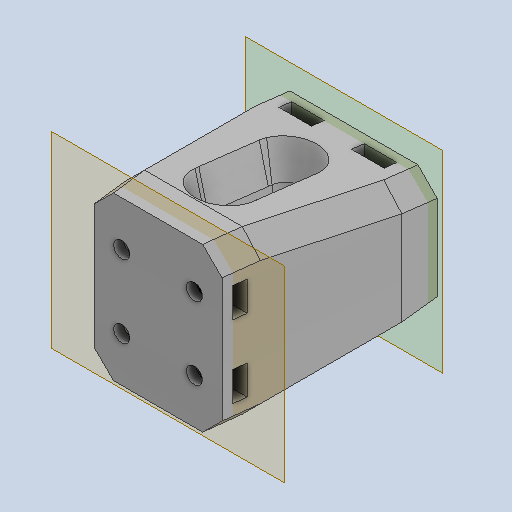
# Autodesk Inventor part: MCP-I
Saved by Autodesk Inventor 2026 (Build 300175050, 175E)
## iProperties
Created: 2025-12-08
Part Number: MCP-I
Material: Genérico
Document SubType Name: Modeling
Designer: user
Density: 1 g/cm^3
Appearance: Gris claro
Mass: 12.7013 g
Surface Area: 55.8888 cm^2
Volume: 12.7013 cm^3
Author: user
Autodesk Inventor part; units mm, degrees
ref_plane "YZ Plane" through (0, 0, 0) normal (1, 0, 0) x (0, 1, 0)
ref_plane "XZ Plane" through (0, 0, 0) normal (0, 1, 0) x (-1, 0, 0)
ref_plane "XY Plane" through (0, 0, 0) normal (0, 0, 1) x (1, 0, 0)
sketch "Boceto1" plane through (0, 0, 0) normal (0, 0, 1) x (1, 0, 0)
  line L0 (-9.8, -13.3) -> (-9.8, 13.3) construction
  line L1 (9.8, 13.3) -> (-9.8, 13.3) construction
  line L2 (9.8, 13.3) -> (9.8, -13.3) construction
  line L3 (-9.8, -13.3) -> (9.8, -13.3) construction
  circle A0 centre (-8, -8) radius 0.8 construction
  circle A1 centre (8, 8) radius 0.8 construction
  circle A2 centre (-8, 8) radius 0.8 construction
  circle A3 centre (0, 0) radius 4 construction
  circle A4 centre (0, -6) radius 1.025 construction
  circle A5 centre (-6, 0) radius 1.025 construction
  circle A6 centre (0, 6) radius 1.025 construction
  circle A7 centre (6, 0) radius 1.025 construction
  circle A8 centre (-5.6569, -5.6569) radius 1.025 construction
  circle A9 centre (-5.6569, 5.6569) radius 1.025 construction
  circle A10 centre (5.6569, 5.6569) radius 1.025 construction
  circle A11 centre (5.6569, -5.6569) radius 1.025 construction
  circle A12 centre (3, -9) radius 1.025 construction
  circle A13 centre (-3, -9) radius 1.025 construction
  circle A14 centre (3, 9) radius 1.025 construction
  circle A15 centre (-3, 9) radius 1.025 construction
  circle A16 centre (8, -8) radius 0.8 construction
  circle A17 centre (5.6569, 5.6569) radius 1.25
  circle A18 centre (5.6569, -5.6569) radius 1.25
  circle A19 centre (-5.6569, -5.6569) radius 1.25
  circle A20 centre (-5.6569, 5.6569) radius 1.25
  line L4 (16.5, -9.7) -> (16.5, 9.7) construction
  line L5 (16.5, 9.7) -> (-16.5, 9.7) construction
  line L6 (-16.5, -9.7) -> (16.5, -9.7) construction
  line L7 (-16.5, -9.7) -> (-16.5, 9.7) construction
  arc A21 (3.8297, -1.1547) -> (3.8297, 1.1547) centre (0, 0) ccw construction
  line L8 (3.8297, -1.1547) -> (4, -1.1547) construction
  line L9 (4, -1.1547) -> (4.7835, -1.6071) construction
  line L10 (4.7835, -1.6071) -> (4.8435, -1.5031) construction
  line L11 (4.8435, -1.5031) -> (5.2765, -1.7531) construction
  line L12 (5.2765, -1.7531) -> (5.2165, -1.8571) construction
  line L13 (5.2165, -1.8571) -> (6, -2.3094) construction
  line L14 (6, -2.3094) -> (8, -1.1547) construction
  line L15 (8, -1.1547) -> (8, -0.25) construction
  line L16 (8, -0.25) -> (7.88, -0.25) construction
  line L17 (7.88, -0.25) -> (7.88, 0.25) construction
  line L18 (7.88, 0.25) -> (8, 0.25) construction
  line L19 (8, 0.25) -> (8, 1.1547) construction
  line L20 (8, 1.1547) -> (6, 2.3094) construction
  line L21 (6, 2.3094) -> (5.2165, 1.8571) construction
  line L22 (5.2165, 1.8571) -> (5.2765, 1.7531) construction
  line L23 (5.2765, 1.7531) -> (4.8435, 1.5031) construction
  line L24 (4.8435, 1.5031) -> (4.7835, 1.6071) construction
  line L25 (4.7835, 1.6071) -> (4, 1.1547) construction
  line L26 (4, 1.1547) -> (3.8297, 1.1547) construction
  circle A22 centre (6, 0) radius 1.025 construction
  arc A23 (3.8297, -1.1547) -> (3.8297, 1.1547) centre (0, 0) ccw construction
  line L27 (3.8297, -1.1547) -> (4, -1.1547) construction
  line L28 (4, -1.1547) -> (4.7835, -1.6071) construction
  line L29 (4.7835, -1.6071) -> (4.8435, -1.5031) construction
  line L30 (4.8435, -1.5031) -> (5.2765, -1.7531) construction
  line L31 (5.2765, -1.7531) -> (5.2165, -1.8571) construction
  line L32 (5.2165, -1.8571) -> (6, -2.3094) construction
  line L33 (6, -2.3094) -> (8, -1.1547) construction
  line L34 (8, -1.1547) -> (8, -0.25) construction
  line L35 (8, -0.25) -> (7.88, -0.25) construction
  line L36 (7.88, -0.25) -> (7.88, 0.25) construction
  line L37 (7.88, 0.25) -> (8, 0.25) construction
  line L38 (8, 0.25) -> (8, 1.1547) construction
  line L39 (8, 1.1547) -> (6, 2.3094) construction
  line L40 (6, 2.3094) -> (5.2165, 1.8571) construction
  line L41 (5.2165, 1.8571) -> (5.2765, 1.7531) construction
  line L42 (5.2765, 1.7531) -> (4.8435, 1.5031) construction
  line L43 (4.8435, 1.5031) -> (4.7835, 1.6071) construction
  line L44 (4.7835, 1.6071) -> (4, 1.1547) construction
  line L45 (4, 1.1547) -> (3.8297, 1.1547) construction
  circle A24 centre (6, 0) radius 1.025 construction
  line L46 (3.3475, 5.6569) -> (4.5022, 7.6569) construction
  line L47 (4.5022, 7.6569) -> (6.8116, 7.6569) construction
  line L48 (6.8116, 7.6569) -> (7.9663, 5.6569) construction
  line L49 (7.9663, 5.6569) -> (6.8116, 3.6569) construction
  line L50 (6.8116, 3.6569) -> (4.5022, 3.6569) construction
  line L51 (4.5022, 3.6569) -> (3.3475, 5.6569) construction
  line L52 (12.9663, -12.6569) -> (-12.9663, -12.6569)
  line L53 (-12.9663, -12.6569) -> (-12.9663, 12.6569)
  line L54 (-12.9663, 12.6569) -> (12.9663, 12.6569)
  line L55 (12.9663, 12.6569) -> (12.9663, -12.6569)
  line L56 (12.9663, -12.6569) -> (-12.9663, 12.6569) construction
  line L57 (-12.9663, -12.6569) -> (12.9663, 12.6569) construction
  line L58 (3.6569, -4.5022) -> (5.6569, -3.3475) construction
  line L59 (5.6569, -3.3475) -> (7.6569, -4.5022) construction
  line L60 (7.6569, -4.5022) -> (7.6569, -6.8116) construction
  line L61 (7.6569, -6.8116) -> (5.6569, -7.9663) construction
  line L62 (5.6569, -7.9663) -> (3.6569, -6.8116) construction
  line L63 (3.6569, -6.8116) -> (3.6569, -4.5022) construction
  point P0 (0, 0)
  point P1 (9.8, -9.7)
  point P2 (9.8, 9.7)
  point P3 (-9.8, -9.7)
  point P4 (-9.8, 9.7)
  point P5 (16.5, 9.7)
extrude "Extrusión1" add sketch "Boceto1" along normal mid plane 30.507
ref_plane "Plano de trabajo1" through (0, 0, 13.7535) normal (0, 0, 1) x (1, 0, 0)
sketch "Boceto2" plane through (0, 0, 13.7535) normal (0, 0, -1) x (-1, 0, 0)
  circle A0 centre (-5.6569, 5.6569) radius 1.25 projected
  circle A1 centre (-5.6569, -5.6569) radius 1.25 projected
  circle A2 centre (5.6569, -5.6569) radius 1.25 projected
  circle A3 centre (5.6569, 5.6569) radius 1.25 projected
  line L0 (-12.9663, 12.6569) -> (-12.9663, -12.6569) projected
  line L1 (-12.9663, -12.6569) -> (12.9663, -12.6569) projected
  line L2 (12.9663, -12.6569) -> (12.9663, 12.6569) projected
  line L3 (12.9663, 12.6569) -> (-12.9663, 12.6569) projected
  arc A4 (-3.8297, 1.1547) -> (-3.8297, -1.1547) centre (0, 0) ccw construction
  line L4 (-3.8297, -1.1547) -> (-4, -1.1547) construction
  line L5 (-4, -1.1547) -> (-4.7835, -1.6071) construction
  line L6 (-4.7835, -1.6071) -> (-4.8435, -1.5031) construction
  line L7 (-4.8435, -1.5031) -> (-5.2765, -1.7531) construction
  line L8 (-5.2765, -1.7531) -> (-5.2165, -1.8571) construction
  line L9 (-5.2165, -1.8571) -> (-6, -2.3094) construction
  line L10 (-6, -2.3094) -> (-8, -1.1547) construction
  line L11 (-8, -1.1547) -> (-8, -0.25) construction
  line L12 (-8, -0.25) -> (-7.88, -0.25) construction
  line L13 (-7.88, -0.25) -> (-7.88, 0.25) construction
  line L14 (-7.88, 0.25) -> (-8, 0.25) construction
  line L15 (-8, 0.25) -> (-8, 1.1547) construction
  line L16 (-8, 1.1547) -> (-6, 2.3094) construction
  line L17 (-6, 2.3094) -> (-5.2165, 1.8571) construction
  line L18 (-5.2165, 1.8571) -> (-5.2765, 1.7531) construction
  line L19 (-5.2765, 1.7531) -> (-4.8435, 1.5031) construction
  line L20 (-4.8435, 1.5031) -> (-4.7835, 1.6071) construction
  line L21 (-4.7835, 1.6071) -> (-4, 1.1547) construction
  line L22 (-4, 1.1547) -> (-3.8297, 1.1547) construction
  circle A5 centre (-6, 0) radius 1.025 construction
  line L23 (-3.6569, -6.8116) -> (-5.6569, -7.9663)
  line L24 (-5.6569, -7.9663) -> (-7.6569, -6.8116)
  line L25 (-7.6569, -6.8116) -> (-7.6569, -4.5022)
  line L26 (-7.6569, -4.5022) -> (-5.6569, -3.3475)
  line L27 (-5.6569, -3.3475) -> (-3.6569, -4.5022)
  line L28 (-3.6569, -4.5022) -> (-3.6569, -6.8116)
  line L29 (-5.6569, -7.9663) -> (-12.9663, -7.9663)
  line L30 (-12.9663, -7.9663) -> (-12.9663, -3.3475)
  line L31 (-12.9663, -3.3475) -> (-5.6569, -3.3475)
  line L32 (-12.9663, 0) -> (12.9663, 0) construction
  line L33 (0, -12.6569) -> (0, 12.6569) construction
  circle A6 centre (-5.6569, 5.6569) radius 1.25
  line L34 (-3.6569, 6.8116) -> (-5.6569, 7.9663)
  line L35 (-5.6569, 7.9663) -> (-7.6569, 6.8116)
  line L36 (-7.6569, 6.8116) -> (-7.6569, 4.5022)
  line L37 (-7.6569, 4.5022) -> (-5.6569, 3.3475)
  line L38 (-5.6569, 3.3475) -> (-3.6569, 4.5022)
  line L39 (-3.6569, 4.5022) -> (-3.6569, 6.8116)
  line L40 (-5.6569, 7.9663) -> (-12.9663, 7.9663)
  line L41 (-12.9663, 7.9663) -> (-12.9663, 3.3475)
  line L42 (-12.9663, 3.3475) -> (-5.6569, 3.3475)
  circle A7 centre (5.6569, 5.6569) radius 1.25
  circle A8 centre (5.6569, -5.6569) radius 1.25
  line L43 (3.6569, -6.8116) -> (5.6569, -7.9663)
  line L44 (5.6569, -7.9663) -> (7.6569, -6.8116)
  line L45 (7.6569, -6.8116) -> (7.6569, -4.5022)
  line L46 (7.6569, -4.5022) -> (5.6569, -3.3475)
  line L47 (5.6569, -3.3475) -> (3.6569, -4.5022)
  line L48 (3.6569, -4.5022) -> (3.6569, -6.8116)
  line L49 (5.6569, -7.9663) -> (12.9663, -7.9663)
  line L50 (12.9663, -7.9663) -> (12.9663, -3.3475)
  line L51 (12.9663, -3.3475) -> (5.6569, -3.3475)
  circle A9 centre (5.6569, 5.6569) radius 1.25
  line L52 (7.6569, 4.5022) -> (5.6569, 3.3475)
  line L53 (5.6569, 3.3475) -> (3.6569, 4.5022)
  line L54 (7.6569, 6.8116) -> (7.6569, 4.5022)
  line L55 (3.6569, 4.5022) -> (3.6569, 6.8116)
  line L56 (3.6569, 6.8116) -> (5.6569, 7.9663)
  line L57 (5.6569, 7.9663) -> (7.6569, 6.8116)
  line L58 (12.9663, 3.3475) -> (5.6569, 3.3475)
  line L59 (12.9663, 7.9663) -> (12.9663, 3.3475)
  line L60 (5.6569, 7.9663) -> (12.9663, 7.9663)
  dimension "d120" = 4.6188
  dimension "d121" = 4.6188
  constraints: 76 end point, 31 symmetric about line, 4 centre point, 4 coincident, 4 midpoint, 2 parallel, 2 perpendicular, 2 vertical, 1 collinear, 1 horizontal, 17 other
  measures "d120" distance of L16.end L9.end
  measures "d121" distance of L26.end L23.end
extrude "Extrusión2" cut sketch "Boceto2" along normal blind 2 contours A0 | A1 | A2 | A3 | L40 L35 L36 L37 L42 L0 | L34 L39 L38 L37 L36 L35 | L2 L58 L52 L54 L57 L60 | L31 L26 L25 L24 L29 L0 | L57 L54 L52 L53 L55 L56 | L27 L28 L23 L24 L25 L26 | L2 L49 L44 L45 L46 L51 | L46 L45 L44 L43 L48 L47
mirror "Simetría2" [suppressed]
ref_plane "Plano de trabajo2" through (0, 0, -13.7535) normal (0, 0, -1) x (-1, 0, 0)
sketch "Boceto7" plane through (0, 0, -13.7535) normal (0, 0, -1) x (-1, 0, 0)
  circle A0 centre (-5.6569, 5.6569) radius 1.25 projected
  circle A1 centre (-5.6569, -5.6569) radius 1.25 projected
  circle A2 centre (5.6569, -5.6569) radius 1.25 projected
  circle A3 centre (5.6569, 5.6569) radius 1.25 projected
  line L0 (-12.9663, -12.6569) -> (-12.9663, 12.6569) projected
  line L1 (-12.9663, 12.6569) -> (12.9663, 12.6569) projected
  line L2 (12.9663, 12.6569) -> (12.9663, -12.6569) projected
  line L3 (12.9663, -12.6569) -> (-12.9663, -12.6569) projected
  arc A4 (-1.1547, -3.8297) -> (1.1547, -3.8297) centre (0, 0) ccw construction
  line L4 (-1.1547, -3.8297) -> (-1.1547, -4) construction
  line L5 (-1.1547, -4) -> (-1.6071, -4.7835) construction
  line L6 (-1.6071, -4.7835) -> (-1.5031, -4.8435) construction
  line L7 (-1.5031, -4.8435) -> (-1.7531, -5.2765) construction
  line L8 (-1.7531, -5.2765) -> (-1.8571, -5.2165) construction
  line L9 (-1.8571, -5.2165) -> (-2.3094, -6) construction
  line L10 (-2.3094, -6) -> (-1.1547, -8) construction
  line L11 (-1.1547, -8) -> (-0.25, -8) construction
  line L12 (-0.25, -8) -> (-0.25, -7.88) construction
  line L13 (-0.25, -7.88) -> (0.25, -7.88) construction
  line L14 (0.25, -7.88) -> (0.25, -8) construction
  line L15 (0.25, -8) -> (1.1547, -8) construction
  line L16 (1.1547, -8) -> (2.3094, -6) construction
  line L17 (2.3094, -6) -> (1.8571, -5.2165) construction
  line L18 (1.8571, -5.2165) -> (1.7531, -5.2765) construction
  line L19 (1.7531, -5.2765) -> (1.5031, -4.8435) construction
  line L20 (1.5031, -4.8435) -> (1.6071, -4.7835) construction
  line L21 (1.6071, -4.7835) -> (1.1547, -4) construction
  line L22 (1.1547, -4) -> (1.1547, -3.8297) construction
  circle A5 centre (0, -6) radius 1.025 construction
  line L23 (4.5022, -7.6569) -> (3.3475, -5.6569) construction
  line L24 (3.3475, -5.6569) -> (4.5022, -3.6569) construction
  line L25 (4.5022, -3.6569) -> (6.8116, -3.6569) construction
  line L26 (6.8116, -3.6569) -> (7.9663, -5.6569) construction
  line L27 (7.9663, -5.6569) -> (6.8116, -7.6569) construction
  line L28 (6.8116, -7.6569) -> (4.5022, -7.6569) construction
  line L29 (4.3867, -7.8569) -> (3.1165, -5.6569)
  line L30 (3.1165, -5.6569) -> (4.3867, -3.4569)
  line L31 (4.3867, -3.4569) -> (6.927, -3.4569)
  line L32 (6.927, -3.4569) -> (8.1972, -5.6569)
  line L33 (8.1972, -5.6569) -> (6.927, -7.8569)
  line L34 (6.927, -7.8569) -> (4.3867, -7.8569)
  line L35 (3.1165, -5.6569) -> (3.1165, -12.6569)
  line L36 (3.1165, -12.6569) -> (8.1972, -12.6569)
  line L37 (8.1972, -12.6569) -> (8.1972, -5.6569)
  line L38 (12.9663, 0) -> (-12.9663, 0) construction
  line L39 (0, 12.6569) -> (0, -12.6569) construction
  circle A6 centre (5.6569, 5.6569) radius 1.25
  line L40 (4.5022, 7.6569) -> (3.3475, 5.6569) construction
  line L41 (3.3475, 5.6569) -> (4.5022, 3.6569) construction
  line L42 (4.5022, 3.6569) -> (6.8116, 3.6569) construction
  line L43 (6.8116, 3.6569) -> (7.9663, 5.6569) construction
  line L44 (7.9663, 5.6569) -> (6.8116, 7.6569) construction
  line L45 (6.8116, 7.6569) -> (4.5022, 7.6569) construction
  line L46 (4.3867, 7.8569) -> (3.1165, 5.6569)
  line L47 (3.1165, 5.6569) -> (4.3867, 3.4569)
  line L48 (4.3867, 3.4569) -> (6.927, 3.4569)
  line L49 (6.927, 3.4569) -> (8.1972, 5.6569)
  line L50 (8.1972, 5.6569) -> (6.927, 7.8569)
  line L51 (6.927, 7.8569) -> (4.3867, 7.8569)
  line L52 (3.1165, 5.6569) -> (3.1165, 12.6569)
  line L53 (3.1165, 12.6569) -> (8.1972, 12.6569)
  line L54 (8.1972, 12.6569) -> (8.1972, 5.6569)
  circle A7 centre (-5.6569, -5.6569) radius 1.25
  circle A8 centre (-5.6569, 5.6569) radius 1.25
  line L55 (-12.9663, -12.6569) -> (12.9663, -12.6569)
  line L56 (-4.5022, -7.6569) -> (-3.3475, -5.6569) construction
  line L57 (-3.3475, -5.6569) -> (-4.5022, -3.6569) construction
  line L58 (-4.5022, -3.6569) -> (-6.8116, -3.6569) construction
  line L59 (-6.8116, -3.6569) -> (-7.9663, -5.6569) construction
  line L60 (-7.9663, -5.6569) -> (-6.8116, -7.6569) construction
  line L61 (-6.8116, -7.6569) -> (-4.5022, -7.6569) construction
  line L62 (-4.3867, -7.8569) -> (-3.1165, -5.6569)
  line L63 (-3.1165, -5.6569) -> (-4.3867, -3.4569)
  line L64 (-4.3867, -3.4569) -> (-6.927, -3.4569)
  line L65 (-6.927, -3.4569) -> (-8.1972, -5.6569)
  line L66 (-8.1972, -5.6569) -> (-6.927, -7.8569)
  line L67 (-6.927, -7.8569) -> (-4.3867, -7.8569)
  line L68 (-3.1165, -5.6569) -> (-3.1165, -12.6569)
  line L69 (-3.1165, -12.6569) -> (-8.1972, -12.6569)
  line L70 (-8.1972, -12.6569) -> (-8.1972, -5.6569)
  circle A9 centre (-5.6569, 5.6569) radius 1.25
  line L71 (-3.1165, 5.6569) -> (-4.3867, 3.4569)
  line L72 (-4.5022, 7.6569) -> (-3.3475, 5.6569) construction
  line L73 (-6.8116, 7.6569) -> (-4.5022, 7.6569) construction
  line L74 (-6.927, 7.8569) -> (-4.3867, 7.8569)
  line L75 (-4.3867, 7.8569) -> (-3.1165, 5.6569)
  line L76 (-7.9663, 5.6569) -> (-6.8116, 7.6569) construction
  line L77 (-8.1972, 5.6569) -> (-6.927, 7.8569)
  line L78 (-3.1165, 5.6569) -> (-3.1165, 12.6569)
  line L79 (-8.1972, 12.6569) -> (-8.1972, 5.6569)
  line L80 (-3.1165, 12.6569) -> (-8.1972, 12.6569)
  line L81 (-4.5022, 3.6569) -> (-6.8116, 3.6569) construction
  line L82 (-4.3867, 3.4569) -> (-6.927, 3.4569)
  line L83 (-6.8116, 3.6569) -> (-7.9663, 5.6569) construction
  line L84 (-6.927, 3.4569) -> (-8.1972, 5.6569)
  line L85 (-3.3475, 5.6569) -> (-4.5022, 3.6569) construction
  point P0 (0, 0)
  point P1 (8.1972, -12.6569)
  point P2 (8.1972, 12.6569)
  point P3 (3.1165, 12.6569)
  point P4 (-8.1972, -12.6569)
  point P5 (-3.1165, -12.6569)
  point P6 (-3.1165, 12.6569)
  point P7 (-8.1972, 12.6569)
  dimension "d123" = 4.6188
  dimension "d124" = 0.2
  dimension "d125" = 4.6188
  constraints: 126 end point, 51 symmetric about line, 4 centre point, 4 coincident, 4 midpoint, 3 parallel, 2 perpendicular, 1 collinear, 1 horizontal, 22 other
  measures "d123" distance of L9.end L16.end
  measures "d124" distance between parallel lines of L28 L34
  measures "d125" distance of L26.end L23.end
extrude "Extrusión6" cut sketch "Boceto7" against normal blind 2 contours A0 | A1 | A2 | A3 | L70 L66 L67 L62 L68 L3 | L1 L78 L75 L74 L77 L79 | L65 L64 L63 L62 L67 L66 | L77 L74 L75 L71 L82 L84 | L35 L29 L34 L33 L37 L3 | L1 L54 L50 L51 L46 L52 | L30 L31 L32 L33 L34 L29 | L46 L51 L50 L49 L48 L47
chamfer "Chaflán2" distance 3 distance2 25 2 edges at (12.9663, 0, 15.2535) (-12.9663, 0, 15.2535) measured on face at (-12.4663, 0, 15.2535) measured on face at (12.4663, 0, 15.2535)
chamfer "Chaflán5" distance 3 distance2 25 2 edges at (0, -12.6569, -15.2535) (0, 12.6569, -15.2535) measured on face at (0, 12.1569, -15.2535) measured on face at (0, -12.1569, -15.2535)
chamfer "Chaflán6" distance 3 angle 45 12 edges at (-11.7967, -11.4873, 0) (-11.7967, 11.4873, 0) (11.7967, 11.4873, 0) (11.7967, -11.4873, 0) (12.9663, -9.9873, -12.5) (12.9663, 9.9873, -12.5) (10.2967, -12.6569, 12.5) (-10.2967, -12.6569, 12.5) (10.2967, 12.6569, 12.5) (-12.9663, -9.9873, -12.5) (-10.2967, 12.6569, 12.5) (-12.9663, 9.9873, -12.5)
sketch "Boceto5" plane through (0, 0, 0) normal (0, 1, 0) x (-1, 0, 0)
  line L0 (0, -5) -> (0, 5) construction
  line L1 (2.5, -5) -> (2.5, 5)
  line L2 (-2.5, 5) -> (-2.5, -5)
  arc A0 (-2.5, -5) -> (2.5, -5) centre (0, -5) ccw
  arc A1 (2.5, 5) -> (-2.5, 5) centre (0, 5) ccw
  point P0 (0, 0)
  dimension "d97" = 5
  dimension "d106" = 15
  constraints: 8 end point, 4 point on circle, 4 tangent, 2 centre point, 1 midpoint, 1 parallel, 1 vertical
  measures "d97" diameter of A1
extrude "Extrusión4" cut sketch "Boceto5" along normal through all both and the other way through all
chamfer "Chaflán7" distance 2 distance2 5 4 edges at (2.5, 11.4873, 0) (0, 12.3873, 7.5) (-2.5, 11.4873, 0) (0, 10.5873, -7.5) measured on face at (3, 11.4873, 0) measured on face at (0, 12.4468, 7.9964) measured on face at (-3, 11.4873, 0) measured on face at (0, 10.5277, -7.9964)
chamfer "Chaflán8" distance 2 distance2 5 4 edges at (2.5, -11.4873, 0) (0, -10.5873, -7.5) (-2.5, -11.4873, 0) (0, -12.3873, 7.5) measured on face at (3, -11.4873, 0) measured on face at (0, -10.5277, -7.9964) measured on face at (0, -12.4468, 7.9964) measured on face at (-3, -11.4873, 0)
sketch "Boceto6" plane through (16.5, -10.3, -15.2535) normal (0, 0, -1) x (-1, 0, 0)
  line L0 (0, 20.6) -> (33, 20.6) construction
  line L1 (33, 20.6) -> (33, 0) construction
  line L2 (33, 0) -> (0, 0) construction
  line L3 (0, 0) -> (0, 20.6) construction
  circle A0 centre (22.1569, 15.9569) radius 1.25 projected
  circle A1 centre (22.1569, 4.6431) radius 1.25 projected
  circle A2 centre (10.8431, 4.6431) radius 1.25 projected
  circle A3 centre (10.8431, 15.9569) radius 1.25 projected
  line L4 (8.3028, 0.4631) -> (13.3835, 0.4631) construction
  line L5 (8.3028, 4.6431) -> (8.3028, 0.4631) construction
  line L6 (9.573, 6.8431) -> (8.3028, 4.6431) construction
  line L7 (12.1133, 6.8431) -> (9.573, 6.8431) construction
  line L8 (13.3835, 4.6431) -> (12.1133, 6.8431) construction
  line L9 (13.3835, 0.4631) -> (13.3835, 4.6431) construction
  circle A4 centre (10.8431, 4.6431) radius 1.25 construction
  line L10 (6.5337, 19.9569) -> (26.4663, 19.9569) projected
  line L11 (26.4663, 19.9569) -> (29.4663, 16.9353) projected
  line L12 (29.4663, 16.9353) -> (29.4663, 3.6647) projected
  line L13 (29.4663, 3.6647) -> (26.4663, 0.6431) projected
  line L14 (26.4663, 0.6431) -> (6.5337, 0.6431) projected
  line L15 (6.5337, 0.6431) -> (3.5337, 3.6647) projected
  line L16 (3.5337, 3.6647) -> (3.5337, 16.9353) projected
  line L17 (3.5337, 16.9353) -> (6.5337, 19.9569) projected
  line L18 (12.3833, 8.3) -> (11.3849, 8.3)
  line L19 (11.3849, 8.3) -> (11.3849, 10.9515)
  line L20 (11.3849, 10.9515) -> (10.6588, 9.24)
  line L21 (10.6588, 9.24) -> (9.9716, 9.24)
  line L22 (9.9716, 9.24) -> (9.2455, 10.9515)
  line L23 (9.2455, 10.9515) -> (9.2455, 8.3)
  line L24 (9.2455, 8.3) -> (8.299, 8.3)
  line L25 (8.299, 8.3) -> (8.299, 12.3)
  line L26 (8.299, 12.3) -> (9.4562, 12.3)
  line L27 (9.4562, 12.3) -> (10.3444, 10.3259)
  line L28 (10.3444, 10.3259) -> (11.2261, 12.3)
  line L29 (11.2261, 12.3) -> (12.3833, 12.3)
  line L30 (12.3833, 12.3) -> (12.3833, 8.3)
  spline S0 degree 2 poles (14.9376, 8.2222) (14.0365, 8.2222) (12.9797, 9.3113) (12.9797, 10.2968) knots 0 0 0 1 2 2 2
  spline S1 degree 2 poles (12.9797, 10.2968) (12.9797, 11.2465) (14.0397, 12.3778) (14.9408, 12.3778) knots 0 0 0 1 2 2 2
  spline S2 degree 2 poles (14.9408, 12.3778) (15.1775, 12.3778) (15.56, 12.3227) (15.735, 12.2773) knots 0 0 0 1 2 2 2
  spline S3 degree 2 poles (15.735, 12.2773) (15.8712, 12.2352) (16.1921, 12.0958) (16.2925, 12.0439) knots 0 0 0 1 2 2 2
  line L31 (16.2925, 12.0439) -> (16.2925, 11.0909)
  line L32 (16.2925, 11.0909) -> (16.1921, 11.0909)
  spline S4 degree 2 poles (16.1921, 11.0909) (16.1175, 11.1558) (15.8971, 11.3373) (15.7577, 11.4216) knots 0 0 0 1 2 2 2
  spline S5 degree 2 poles (15.7577, 11.4216) (15.6183, 11.5091) (15.2844, 11.629) (15.0997, 11.629) knots 0 0 0 1 2 2 2
  spline S6 degree 2 poles (15.0997, 11.629) (14.8825, 11.629) (14.5227, 11.4929) (14.3574, 11.3211) knots 0 0 0 1 2 2 2
  spline S7 degree 2 poles (14.3574, 11.3211) (14.2083, 11.1687) (14.017, 10.6468) (14.017, 10.2935) knots 0 0 0 1 2 2 2
  spline S8 degree 2 poles (14.017, 10.2935) (14.017, 9.9207) (14.2147, 9.4118) (14.3768, 9.2562) knots 0 0 0 1 2 2 2
  spline S9 degree 2 poles (14.3768, 9.2562) (14.5324, 9.1039) (14.9149, 8.971) (15.1062, 8.971) knots 0 0 0 1 2 2 2
  spline S10 degree 2 poles (15.1062, 8.971) (15.3039, 8.971) (15.6637, 9.1039) (15.7869, 9.1849) knots 0 0 0 1 2 2 2
  spline S11 degree 2 poles (15.7869, 9.1849) (15.923, 9.266) (16.1272, 9.4378) (16.2018, 9.5058) knots 0 0 0 1 2 2 2
  line L33 (16.2018, 9.5058) -> (16.2925, 9.5058)
  line L34 (16.2925, 9.5058) -> (16.2925, 8.5658)
  spline S12 degree 2 poles (16.2925, 8.5658) (16.1823, 8.5139) (15.8938, 8.3843) (15.7382, 8.3389) knots 0 0 0 1 2 2 2
  spline S13 degree 2 poles (15.7382, 8.3389) (15.5502, 8.2806) (15.2229, 8.2222) (14.9376, 8.2222) knots 0 0 0 1 2 2 2
  spline S14 degree 2 poles (19.9619, 11.0391) (19.9619, 10.7603) (19.7836, 10.2546) (19.6183, 10.0861) knots 0 0 0 1 2 2 2
  spline S15 degree 2 poles (19.6183, 10.0861) (19.5178, 9.9791) (19.2715, 9.8041) (19.1256, 9.7425) knots 0 0 0 1 2 2 2
  spline S16 degree 2 poles (19.1256, 9.7425) (18.9765, 9.6809) (18.6297, 9.6096) (18.4157, 9.6096) knots 0 0 0 1 2 2 2
  line L35 (18.4157, 9.6096) -> (17.8906, 9.6096)
  line L36 (17.8906, 9.6096) -> (17.8906, 8.3)
  line L37 (17.8906, 8.3) -> (16.8857, 8.3)
  line L38 (16.8857, 8.3) -> (16.8857, 12.3)
  line L39 (16.8857, 12.3) -> (18.4384, 12.3)
  spline S17 degree 2 poles (18.4384, 12.3) (18.782, 12.3) (19.2844, 12.1736) (19.4887, 12.0374) knots 0 0 0 1 2 2 2
  spline S18 degree 2 poles (19.4887, 12.0374) (19.7156, 11.8851) (19.9619, 11.3859) (19.9619, 11.0391) knots 0 0 0 1 2 2 2
  spline S19 degree 2 poles (18.9311, 11.0131) (18.9311, 11.1849) (18.769, 11.428) (18.6588, 11.4734) knots 0 0 0 1 2 2 2
  spline S20 degree 2 poles (18.6588, 11.4734) (18.5162, 11.535) (18.2569, 11.5545) (18.0332, 11.5545) knots 0 0 0 1 2 2 2
  line L40 (18.0332, 11.5545) -> (17.8906, 11.5545)
  line L41 (17.8906, 11.5545) -> (17.8906, 10.3551)
  line L42 (17.8906, 10.3551) -> (17.9619, 10.3551)
  spline S21 degree 2 poles (17.9619, 10.3551) (18.1013, 10.3551) (18.3541, 10.3616) (18.4481, 10.3778) knots 0 0 0 1 2 2 2
  spline S22 degree 2 poles (18.4481, 10.3778) (18.5292, 10.3908) (18.7075, 10.4686) (18.7561, 10.5172) knots 0 0 0 1 2 2 2
  spline S23 degree 2 poles (18.7561, 10.5172) (18.8598, 10.6144) (18.9311, 10.8316) (18.9311, 11.0131) knots 0 0 0 1 2 2 2
  line L43 (22.1596, 9.6938) -> (20.3801, 9.6938)
  line L44 (20.3801, 9.6938) -> (20.3801, 10.4394)
  line L45 (20.3801, 10.4394) -> (22.1596, 10.4394)
  line L46 (22.1596, 10.4394) -> (22.1596, 9.6938)
  line L47 (24.863, 8.3) -> (22.7107, 8.3)
  line L48 (22.7107, 8.3) -> (22.7107, 8.9969)
  line L49 (22.7107, 8.9969) -> (23.2844, 8.9969)
  line L50 (23.2844, 8.9969) -> (23.2844, 11.6031)
  line L51 (23.2844, 11.6031) -> (22.7107, 11.6031)
  line L52 (22.7107, 11.6031) -> (22.7107, 12.3)
  line L53 (22.7107, 12.3) -> (24.863, 12.3)
  line L54 (24.863, 12.3) -> (24.863, 11.6031)
  line L55 (24.863, 11.6031) -> (24.2893, 11.6031)
  line L56 (24.2893, 11.6031) -> (24.2893, 8.9969)
  line L57 (24.2893, 8.9969) -> (24.863, 8.9969)
  line L58 (24.863, 8.9969) -> (24.863, 8.3)
  point P0 (16.5, 10.3)
  point P1 (0, 20.6)
  constraints: 2 coincident, 2 other
extrude "Extrusión5" cut sketch "Boceto6" against normal blind 0.32 contours L18 L19 L20 L21 L22 L23 L24 L25 L26 L27 L28 L29 L30 | S0 S1 S2 S3 L31 L32 S4 S5 S6 S7 S8 S9 S10 S11 L33 L34 S12 S13 | S14 S15 S16 L35 L36 L37 L38 L39 S17 S18 | L43 L44 L45 L46 | L47 L48 L49 L50 L51 L52 L53 L54 L55 L56 L57 L58
